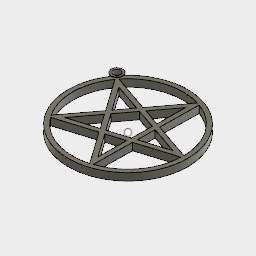
pendant (Autodesk Fusion 360 design; units mm, degrees)
Autodesk Fusion 360 part; units mm, degrees
sketch "草图1" plane through (0, 0, 0) normal (0, 1, 0) x (1, 0, 0)
  point P0 (-25, 10)
sketch "草图2" plane through (0, 0, 0) normal (0, 1, 0) x (1, 0, 0)
  circle A0 centre (-25, 10) radius 40.6099
  line L0 (-13.7666, 45.8931) -> (-29.5688, 24.8235)
  line L1 (-15.0058, 39.2409) -> (-26.584, 23.8033)
  line L2 (-29.5688, 24.8235) -> (-54.4904, 33.3414)
  line L3 (-31.4615, 22.3) -> (-49.7214, 28.541)
  line L4 (-49.7214, 28.541) -> (-38.6172, 12.759)
  line L5 (-31.4615, 22.3) -> (-38.6172, 12.759)
  line L6 (-40.5098, 10.2355) -> (-56.312, -10.8341)
  line L7 (-55.6651, 31.7752) -> (-40.5098, 10.2355)
  line L8 (-28.4766, 21.2798) -> (-36.802, 10.1792)
  line L9 (-38.6947, 7.6557) -> (-50.2729, -7.7819)
  line L10 (-50.2729, -7.7819) -> (-31.8319, -2.0981)
  line L11 (-38.6947, 7.6557) -> (-31.8319, -2.0981)
  line L12 (-30.0168, -4.6779) -> (-14.8615, -26.2176)
  line L13 (-55.1855, -12.4353) -> (-30.0168, -4.6779)
  line L14 (-36.802, 10.1792) -> (-28.8175, -1.169)
  line L15 (-27.0023, -3.7488) -> (-15.8981, -19.5309)
  line L16 (-15.8981, -19.5309) -> (-15.6052, -0.2361)
  line L17 (-28.8175, -1.169) -> (-15.5573, 2.918)
  line L18 (-12.5428, 3.8471) -> (5.8981, 9.5309)
  line L19 (-12.9906, -25.641) -> (-12.5907, 0.693)
  line L20 (-27.0023, -3.7488) -> (-15.6052, -0.2361)
  line L21 (-12.5907, 0.693) -> (12.578, 8.4504)
  line L22 (5.8981, 9.5309) -> (-12.3618, 15.7719)
  line L23 (-15.3466, 16.7921) -> (-28.4766, 21.2798)
  line L24 (12.6077, 10.408) -> (-12.3139, 18.9259)
  line L25 (-15.2987, 19.9461) -> (-26.584, 23.8033)
  line L26 (-15.5573, 2.918) -> (-15.3466, 16.7921)
  line L27 (-15.2987, 19.9461) -> (-15.0058, 39.2409)
  line L28 (-12.5428, 3.8471) -> (-12.3618, 15.7719)
  line L29 (-12.3139, 18.9259) -> (-11.914, 45.2599)
  arc A1 (-13.7666, 45.8931) -> (-54.4904, 33.3414) centre (-25, 10) ccw
  arc A2 (-55.6651, 31.7752) -> (-56.312, -10.8341) centre (-25, 10) ccw
  arc A3 (-55.1855, -12.4353) -> (-14.8615, -26.2176) centre (-25, 10) ccw
  arc A4 (-12.9906, -25.641) -> (12.578, 8.4504) centre (-25, 10) ccw
  arc A5 (12.6077, 10.408) -> (-11.914, 45.2599) centre (-25, 10) ccw
  point P0 (-15.0058, 39.2409)
  point P1 (-50.2729, -7.7819)
  point P2 (5.8981, 9.5309)
  point P3 (-49.7214, 28.541)
  point P4 (-25, 10)
extrude "拉伸1" add sketch "草图2" along normal blind 5 makes body 1
sketch "草图3" plane through (0, 0, 0) normal (0, 1, 0) x (1, 0, 0)
sketch "草图4" plane through (0, 0, 0) normal (0, 1, 0) x (1, 0, 0)
sketch "草图5" plane through (0, 0, 0) normal (0, 1, 0) x (1, 0, 0)
sketch "草图6" plane through (0, 0, 0) normal (0, 1, 0) x (1, 0, 0)
  circle A0 centre (40, -20) radius 2.5
  circle A1 centre (40, -20) radius 4
  dimension "d5" = 5
  dimension "d6" = 8
  measures "d5" diameter of A0
  measures "d6" diameter of A1
extrude "拉伸2" add sketch "草图6" along normal blind 5 separate body makes body 2
move_body "移动1" bodies 2 to x (1, 0, 0) y (0, 1, 0) z (0, 0, 1) at (-108.6235, 0.1986, -28.1984)
move_body "移动2" bodies 2 to x (1, 0, 0) y (0, 1, 0) z (0, 0, 1) at (9.1347, 0, -27.4041)
move_body "移动3" bodies 2 to x (1, 0, 0) y (0, 1, 0) z (0, 0, 1) at (-0.1986, 0, -0.9929)
move_body "移动4" bodies 2 to x (1, 0, 0) y (0, 1, 0) z (0, 0, 1) at (0.3972, 0, 0.7943)
move_body "移动5" bodies 2 to x (1, 0, 0) y (0, 1, 0) z (0, 0, 1) at (0.3972, 0, 0)
move_body "移动6" bodies 2 to x (1, 0, 0) y (0, 1, 0) z (0, 0, 1) at (-0.7943, 0, 0)
move_body "移动7" bodies 2 to x (1, 0, 0) y (0, 1, 0) z (0, 0, 1) at (0.7943, 0, -0.5957)
combine "合并1" operation add target body 1 tool bodies 2
